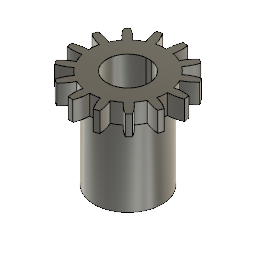
gear14 (Autodesk Fusion 360 design; units mm, degrees)
Autodesk Fusion 360 part; units mm, degrees
sketch "Sketch1" plane through (0, 0, 0) normal (0, 0, 1) x (1, 0, 0)
  line L0 (0, 0) -> (0, -3.17) construction
  line L1 (0, 0) -> (0, 3.17) construction
  line L2 (-0.4, 0) -> (-0.4, 3.1447)
  line L3 (-0.4, 0) -> (-0.4, -3.1447)
  line L4 (0.4, 0) -> (0.4, 3.1447)
  line L5 (0.4, 0) -> (0.4, -3.1447)
  circle A0 centre (0, 0) radius 5.17
  arc A1 (-0.4, 3.1447) -> (-0.4, -3.1447) centre (0, 0) ccw
  arc A2 (0.4, -3.1447) -> (0.4, 3.1447) centre (0, 0) ccw
  dimension "d1" = 6.34
  dimension "d21" = 2
  constraint coincident L0.start L1.start
  constraint vertical L0
  constraint parallel L0 L1
  constraint parallel L1 L4
  constraint parallel L0 L5
  constraint parallel L1 L2
  constraint parallel L0 L3
  constraint coincident L5.end A1
  constraint concentric A1 A2
  measures "d1" diameter of A1
  measures "d21" distance of A0 A2
extrude "Extrude1" add sketch "Sketch1" along normal blind 2
sketch "Sketch2" plane through (0, 0, 2) normal (0, 0, 1) x (-1, 0, 0)
  line L0 (-0.4, 3.1447) -> (-0.4, -3.1447)
  arc A0 (-0.4, 3.1447) -> (-0.4, -3.1447) centre (0, 0) ccw
  line L1 (0.4, -3.1447) -> (0.4, 3.1447)
  arc A1 (0.4, -3.1447) -> (0.4, 3.1447) centre (0, 0) ccw
  circle A2 centre (0, 0) radius 5.17
  circle A3 centre (0, 0) radius 4.17
  circle A4 centre (0, 0) radius 3.1447
  constraint coincident A0.centre A1.centre
  constraint concentric A3 A4
extrude "Extrude2" add sketch "Sketch2" along normal blind 10 contours A2 | A3
sketch "Sketch3" plane through (0, 0, 12) normal (0, 0, 1) x (-1, 0, 0)
  arc A0 (0.4, 3.1191) -> (-0.4, 3.1191) centre (0, 0) ccw
  line L0 (0.4, 3.1191) -> (0.4, 3.1447)
  arc A1 (0.4, -3.1447) -> (0.4, 3.1447) centre (0, 0) ccw
  line L1 (0.4, -3.1447) -> (0.4, -3.1191)
  arc A2 (-0.4, -3.1191) -> (0.4, -3.1191) centre (0, 0) ccw
  line L2 (-0.4, -3.1191) -> (-0.4, -3.1447)
  arc A3 (-0.4, 3.1447) -> (-0.4, -3.1447) centre (0, 0) ccw
  line L3 (-0.4, 3.1447) -> (-0.4, 3.1191)
  circle A4 centre (0, 0) radius 5.17
  circle A5 centre (0, 0) radius 8 construction
  circle A6 centre (0, 0) radius 7 construction
  circle A7 centre (0, 0) radius 5.83 construction
  line L4 (0, 0) -> (0, -8) construction
  line L5 (0, 0) -> (-0.7855, -7.9613) construction
  line L6 (0, 0) -> (-1.571, -7.8442) construction
  arc A8 (-1.1902, -7.911) -> (-0.4082, -7.9896) centre (0, 0) ccw
  arc A9 (-0.4082, -7.9896) -> (0, -5.83) centre (-5.917, -5.83) ccw
  arc A10 (-1.1449, -5.7165) -> (-1.1902, -7.911) centre (4.9671, -6.9406) ccw
  arc A11 (3.0988, -7.3755) -> (2.5295, -5.2526) centre (-2.8015, -7.8199) ccw
  arc A12 (2.3601, -7.644) -> (3.0988, -7.3755) centre (0, 0) ccw
  arc A13 (1.4488, -5.6471) -> (2.3601, -7.644) centre (7.4866, -4.0981) ccw
  arc A14 (5.992, -5.3005) -> (4.5581, -3.6349) centre (0.8689, -8.261) ccw
  arc A15 (5.4429, -5.863) -> (5.992, -5.3005) centre (0, 0) ccw
  arc A16 (3.7555, -4.4593) -> (5.4429, -5.863) centre (8.5233, -0.4439) ccw
  arc A17 (7.6984, -2.1758) -> (5.6838, -1.2973) centre (4.3672, -7.0659) ccw
  arc A18 (7.4478, -2.9208) -> (7.6984, -2.1758) centre (0, 0) ccw
  arc A19 (5.3184, -2.3882) -> (7.4478, -2.9208) centre (7.8718, 3.2982) ccw
  arc A20 (7.8801, 1.3799) -> (5.6838, 1.2973) centre (7.0005, -4.4713) ccw
  arc A21 (7.9775, 0.6) -> (7.8801, 1.3799) centre (0, 0) ccw
  arc A22 (5.8279, 0.1559) -> (7.9775, 0.6) centre (5.6613, 6.387) ccw
  arc A23 (6.501, 4.6623) -> (4.5581, 3.6349) centre (8.2473, -0.9911) ccw
  arc A24 (6.9271, 4.0018) -> (6.501, 4.6623) centre (0, 0) ccw
  arc A25 (5.1831, 2.6691) -> (6.9271, 4.0018) centre (2.3294, 8.2108) ccw
  arc A26 (3.8343, 7.0213) -> (2.5295, 5.2526) centre (7.8606, 2.6854) ccw
  arc A27 (4.5048, 6.6111) -> (3.8343, 7.0213) centre (0, 0) ccw
  arc A28 (3.5118, 4.6536) -> (4.5048, 6.6111) centre (-1.4638, 8.4084) ccw
  arc A29 (0.4082, 7.9896) -> (0, 5.83) centre (5.917, 5.83) ccw
  arc A30 (1.1902, 7.911) -> (0.4082, 7.9896) centre (0, 0) ccw
  arc A31 (1.1449, 5.7165) -> (1.1902, 7.911) centre (-4.9671, 6.9406) ccw
  arc A32 (-3.0988, 7.3755) -> (-2.5295, 5.2526) centre (2.8015, 7.8199) ccw
  arc A33 (-2.3601, 7.644) -> (-3.0988, 7.3755) centre (0, 0) ccw
  arc A34 (-1.4488, 5.6471) -> (-2.3601, 7.644) centre (-7.4866, 4.0981) ccw
  arc A35 (-5.992, 5.3005) -> (-4.5581, 3.6349) centre (-0.8689, 8.261) ccw
  arc A36 (-5.4429, 5.863) -> (-5.992, 5.3005) centre (0, 0) ccw
  arc A37 (-3.7555, 4.4593) -> (-5.4429, 5.863) centre (-8.5233, 0.4439) ccw
  arc A38 (-7.6984, 2.1758) -> (-5.6838, 1.2973) centre (-4.3672, 7.0659) ccw
  arc A39 (-7.4478, 2.9208) -> (-7.6984, 2.1758) centre (0, 0) ccw
  arc A40 (-5.3184, 2.3882) -> (-7.4478, 2.9208) centre (-7.8718, -3.2982) ccw
  arc A41 (-7.8801, -1.3799) -> (-5.6838, -1.2973) centre (-7.0005, 4.4713) ccw
  arc A42 (-7.9775, -0.6) -> (-7.8801, -1.3799) centre (0, 0) ccw
  arc A43 (-5.8279, -0.1559) -> (-7.9775, -0.6) centre (-5.6613, -6.387) ccw
  arc A44 (-6.501, -4.6623) -> (-4.5581, -3.6349) centre (-8.2473, 0.9911) ccw
  arc A45 (-6.9271, -4.0018) -> (-6.501, -4.6623) centre (0, 0) ccw
  arc A46 (-5.1831, -2.6691) -> (-6.9271, -4.0018) centre (-2.3294, -8.2108) ccw
  arc A47 (-3.8343, -7.0213) -> (-2.5295, -5.2526) centre (-7.8606, -2.6854) ccw
  arc A48 (-4.5048, -6.6111) -> (-3.8343, -7.0213) centre (0, 0) ccw
  arc A49 (-3.5118, -4.6536) -> (-4.5048, -6.6111) centre (1.4638, -8.4084) ccw
  arc A50 (-2.5295, -5.2526) -> (-1.1449, -5.7165) centre (0, 0) ccw
  arc A51 (0, -5.83) -> (1.4488, -5.6471) centre (0, 0) ccw
  arc A52 (2.5295, -5.2526) -> (3.7555, -4.4593) centre (0, 0) ccw
  arc A53 (4.5581, -3.6349) -> (5.3184, -2.3882) centre (0, 0) ccw
  arc A54 (5.6838, -1.2973) -> (5.8279, 0.1559) centre (0, 0) ccw
  arc A55 (5.6838, 1.2973) -> (5.1831, 2.6691) centre (0, 0) ccw
  arc A56 (4.5581, 3.6349) -> (3.5118, 4.6536) centre (0, 0) ccw
  arc A57 (2.5295, 5.2526) -> (1.1449, 5.7165) centre (0, 0) ccw
  arc A58 (0, 5.83) -> (-1.4488, 5.6471) centre (0, 0) ccw
  arc A59 (-2.5295, 5.2526) -> (-3.7555, 4.4593) centre (0, 0) ccw
  arc A60 (-4.5581, 3.6349) -> (-5.3184, 2.3882) centre (0, 0) ccw
  arc A61 (-5.6838, 1.2973) -> (-5.8279, -0.1559) centre (0, 0) ccw
  arc A62 (-5.6838, -1.2973) -> (-5.1831, -2.6691) centre (0, 0) ccw
  arc A63 (-4.5581, -3.6349) -> (-3.5118, -4.6536) centre (0, 0) ccw
  dimension "d9" = 16
  dimension "d10" = 14
  dimension "d11" = 11.66
  dimension "d12" = 0.7855
  dimension "d13" = 1.571
  dimension "d14" = 0.786
  dimension "d16" = 360
  dimension "d18" = 360
  constraint coincident A0.centre A1.centre
  constraint concentric A5 A6
  constraint concentric A6 A7
  constraint coincident A5 L4.end
  constraint vertical L4
  constraint coincident A5 L5.end
  constraint coincident A5 L6.end
  constraint coincident L5.end A8
  constraint coincident A5 A8.start
  constraint coincident A5 A8.end
  constraint tangent L4 A9
  constraint coincident A7 A9.end
  constraint coincident L4 A9.end
  constraint tangent L6 A10
  constraint coincident L6 A10.start
  constraint coincident A7 A10.start
  measures "d9" diameter of A5
  measures "d10" diameter of A6
  measures "d11" diameter of A7
  measures "d12" horizontal distance of L4.end L5.end
  measures "d13" horizontal distance of L4.end L6.end
  measures "d14" distance of A8.end A8.start
extrude "Extrude3" add sketch "Sketch3" along normal blind 3 contours A4 | A8 A9 A10 A11 A12 A13 A14 A15 A16 A17 A18 A19 A20 A21 A22 A23 A24 A25 A26 A27 A28 A29 A30 A31 A32 A33 A34 A35 A36 A37 A38 A39 A40 A41 A42 A43 A44 A45 A46 A47 A48 A49 A50 A51 A52 A53 A54 A55 A56 A57 A58 A59 A60 A61 A62 A63
